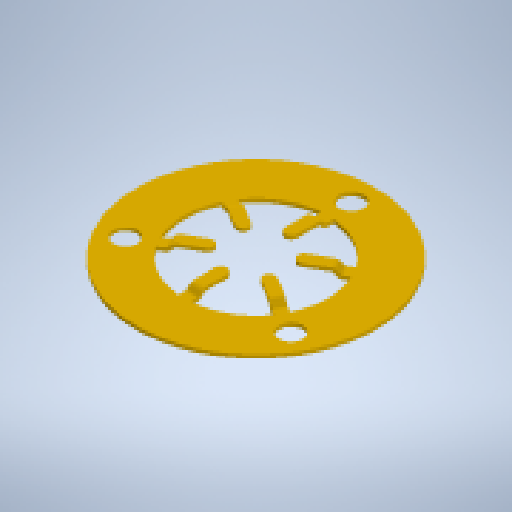
# Autodesk Inventor part: 037
Saved by Autodesk Inventor 2023 (Build 270158000, 158)
## iProperties
Created: 2022-04-25
Part Number: 037
Material: Stainless Steel, Austenitic
Document SubType Name: Sheet Metal
Designer: vmiguel
Density: 8 g/cm^3
Appearance: Gold
Sheet Metal Rule: Default_mm
Author: vmiguel
Autodesk Inventor part; units mm, degrees
ref_plane "YZ Plane" through (0, 0, 0) normal (1, 0, 0) x (0, 1, 0)
ref_plane "XZ Plane" through (0, 0, 0) normal (0, 1, 0) x (-1, 0, 0)
ref_plane "XY Plane" through (0, 0, 0) normal (0, 0, 1) x (1, 0, 0)
sketch "Sketch1" plane through (0, 0, 0) normal (0, 1, 0) x (-1, 0, 0)
  circle A0 centre (0, 0) radius 10
  circle A1 centre (0, -8) radius 1
  circle A2 centre (6.9282, 4) radius 1
  circle A3 centre (-6.9282, 4) radius 1
  circle A4 centre (0, 0) radius 6
  line L0 (0, -2.6) -> (0, -6) construction
  line L1 (-0.75, -2.6) -> (-0.75, -6)
  line L2 (0.75, -6) -> (0.75, -2.6)
  arc A5 (0.75, -2.6) -> (-0.75, -2.6) centre (0, -2.6) ccw
  arc A6 (-0.75, -6) -> (0.75, -6) centre (0, -6) ccw construction
  line L3 (-0.75, -4.3) -> (0.75, -4.3)
  point P0 (0, -4.3)
  point P1 (0.75, -5.9529)
  point P2 (-0.75, -5.9529)
  dimension "d7" = 12
  dimension "d0" = 20
  dimension "d1" = 2
  dimension "d2" = 8
  dimension "d5" = 360
  dimension "d8" = 1.5
  dimension "d9" = 3.4
  measures "d0" diameter of A0
  measures "d1" diameter of A1
  measures "d2" distance of A1.centre point (0, 0)
  measures "d8" distance between parallel lines of L1 L2
  measures "d9" distance of L0.start L0.end
extrude "Plate1" add sketch "Sketch1" along normal blind 0.3
sketch "Sketch2" plane through (0, 0, 0) normal (0, 1, 0) x (-1, 0, 0)
  circle A0 centre (0, 0) radius 6
  line L0 (0.5, -5.5) -> (-0.5, -5.5)
  line L1 (-0.5, -5.5) -> (-0.5, -6.5)
  line L2 (-0.5, -6.5) -> (0.5, -6.5)
  line L3 (0.5, -6.5) -> (0.5, -5.5)
  line L4 (0.5, -5.5) -> (-0.5, -6.5) construction
  line L5 (-0.5, -5.5) -> (0.5, -6.5) construction
  point P0 (0, -6)
  dimension "d17" = 5.5
  dimension "d18" = 1
  dimension "d19" = 1
  measures "d17" distance from line of L0 point (0, 0)
  measures "d18" distance of L0.end L1.end
  measures "d19" distance of L0.start L0.end
sheet face with bend "Face2" sketch "Sketch2" thickness 0.3 toward (0, 1, 0) bend radius 0.3 relief straight relief width 0.3 relief depth 0.15 picked at (-0.0556, -5.6659) contours L1 L0 L3 A0 | A0 L3 L2 L1
bend "Bend1"
sketch "Sketch3" plane through (0.5, 0.3879, -5.2879) normal (0, -0.7071068, 0.7071068) x (1, 0, 0)
  line L0 (-1, 0) -> (0, 0)
  line L1 (0, 0) -> (0, 0.2515)
  line L2 (0, 0.2515) -> (-1, 0.2515)
  line L3 (-1, 0.2515) -> (-1, 0)
  constraints: 6 end point, 1 horizontal, 1 perpendicular, 1 vertical
edge flange "Flange1" height 0.5 angle 45 thickness 0.3 bend radius 0.3 thickness toward (0, -0.7071068, 0.7071068) relief straight relief width 0.3 relief depth 0.15 edges at (0, 0.3, -5.5) wall of the first edge with corners at (-0.5, 0.3879, -5.2879) (0.5, 0.3879, -5.2879) (0.5, 0.5657, -5.1101) (-0.5, 0.5657, -5.1101)
bend "Bend2"
corner "Corner1"
sketch "Sketch4" plane through (-0.5, 0.4414, -4.6858) normal (0, 1, 0) x (-1, 0, 0)
  line L0 (-1, 0) -> (0, 0)
  line L1 (0, 0) -> (0, 2.2515)
  line L2 (0, 2.2515) -> (-1, 2.2515)
  line L3 (-1, 2.2515) -> (-1, 0)
  constraints: 6 end point, 1 horizontal, 1 perpendicular, 1 vertical
edge flange "Flange2" height 2.5 angle 45 thickness 0.3 bend radius 0.3 thickness toward (0, 1, 0) relief straight relief width 0.3 relief depth 0.15 edges at (0, 0.3536, -4.8979) wall of the first edge with corners at (0.5, 0.4414, -4.6858) (-0.5, 0.4414, -4.6858) (-0.5, 0.4414, -2.4343) (0.5, 0.4414, -2.4343)
bend "Bend3"
corner "Corner2"
fillet "Corner Round1" radius 0.5 2 edges at (0.5, 0.5914, -2.4343) (-0.5, 0.5914, -2.4343)
pattern_circular "Circular Pattern1" count 6 over 360 about axis through (0, 0, 0) along (0, 1, 0) of "Face2", "Flange1", "Flange2", "Corner Round1"
equation "\"d16\" = Thickness"
equation "\"d20\" = BendRadius"
equation "\"d21\" = BendReliefWidth"
equation "\"d23\" = MinimumRemnant"
equation "\"d22\" = BendReliefDepth"
equation "\"d24\" = TransitionRadius"
equation "\"d25\" = BendReliefWidth"
equation "\"d26\" = BendReliefDepth"
equation "\"d27\" = MinimumRemnant"
equation "\"d28\" = TransitionRadius"
equation "\"d31\" = BendRadius"
equation "\"d32\" = CornerReliefSize"
equation "\"d33\" = GapSize"
equation "\"d34\" = JacobiRadiusSize"
equation "\"d35\" = BendReliefWidth"
equation "\"d36\" = BendReliefDepth"
equation "\"d37\" = MinimumRemnant"
equation "\"d38\" = TransitionRadius"
equation "\"d41\" = BendRadius"
equation "\"d42\" = CornerReliefSize"
equation "\"d43\" = GapSize"
equation "\"d44\" = JacobiRadiusSize"
equation "\"BendRadius\" = Thickness"
equation "\"BendReliefWidth\" = Thickness"
equation "\"BendReliefDepth\" = 0.5 * Thickness"
equation "\"CornerReliefSize\" = 4 * Thickness"
equation "\"MinimumRemnant\" = 2 * Thickness"
equation "\"TransitionRadius\" = BendRadius"
equation "\"JacobiRadiusSize\" = BendRadius"
equation "\"GapSize\" = Thickness"
equation "\"Thickness\" = 0.3"
body "Solid2"
